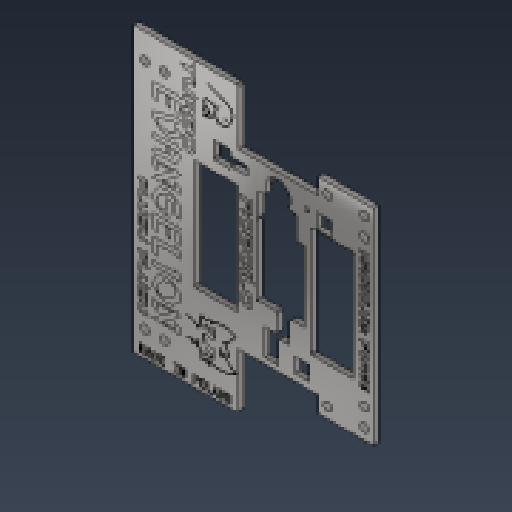
# Autodesk Inventor part: ceil
Saved by Autodesk Inventor 2026.2 (Build 302298010, 298A)
## iProperties
Created: 2026-05-14
Part Number: ceil
Material: Steel, Alloy
Document SubType Name: Modeling
Designer: szymo
Density: 7.73 g/cm^3
Appearance: Semi-Polished
Author: szymo
Autodesk Inventor part; units mm, degrees
(part 1 of 7)
ref_plane "YZ Plane" through (0, 0, 0) normal (1, 0, 0) x (0, 1, 0)
ref_plane "XZ Plane" through (0, 0, 0) normal (0, 1, 0) x (-1, 0, 0)
ref_plane "XY Plane" through (0, 0, 0) normal (0, 0, 1) x (1, 0, 0)
sketch "Katze" plane through (0, 0, 0) normal (0, 0, 1) x (1, 0, 0)
  line L0 (230.7163, -61.7099) -> (230.2113, -62.1007)
  line L1 (230.2113, -62.1007) -> (229.7885, -62.4476)
  line L2 (229.7885, -62.4476) -> (229.4229, -62.7723)
  line L3 (229.4229, -62.7723) -> (229.0894, -63.0967)
  line L4 (229.0894, -63.0967) -> (228.5914, -63.6396)
  line L5 (228.5914, -63.6396) -> (228.3777, -63.9055)
  line L6 (228.3777, -63.9055) -> (228.1831, -64.174)
  line L7 (228.1831, -64.174) -> (228.0044, -64.45)
  line L8 (228.0044, -64.45) -> (227.8384, -64.7383)
  line L9 (227.8384, -64.7383) -> (227.5311, -65.3713)
  line L10 (227.5311, -65.3713) -> (227.3292, -65.8056)
  line L11 (227.3292, -65.8056) -> (227.2039, -65.7151)
  line L12 (227.2039, -65.7151) -> (226.9329, -65.4703)
  line L13 (226.9329, -65.4703) -> (226.5687, -65.1387)
  line L14 (226.5687, -65.1387) -> (226.2195, -64.8603)
  line L15 (226.2195, -64.8603) -> (225.8775, -64.6297)
  line L16 (225.8775, -64.6297) -> (225.5347, -64.4416)
  line L17 (225.5347, -64.4416) -> (225.1793, -64.2897)
  line L18 (225.1793, -64.2897) -> (224.8232, -64.1835)
  line L19 (224.8232, -64.1835) -> (224.4342, -64.1159)
  line L20 (224.4342, -64.1159) -> (223.9802, -64.0797)
  line L21 (223.9802, -64.0797) -> (223.4544, -64.053)
  line L22 (223.4544, -64.053) -> (223.4773, -64.4111)
  line L23 (223.4773, -64.4111) -> (223.5225, -64.766)
  line L24 (223.5225, -64.766) -> (223.6106, -65.1265)
  line L25 (223.6106, -65.1265) -> (223.7387, -65.4827)
  line L26 (223.7387, -65.4827) -> (223.904, -65.8247)
  line L27 (223.904, -65.8247) -> (223.8877, -65.8497)
  line L28 (223.8877, -65.8497) -> (223.8303, -65.8894)
  line L29 (223.8303, -65.8894) -> (223.6435, -65.9885)
  line L30 (223.6435, -65.9885) -> (223.4459, -66.0733)
  line L31 (223.4459, -66.0733) -> (223.3401, -66.0952)
  line L32 (223.3401, -66.0952) -> (221.4618, -63.5691)
  line L33 (221.4618, -63.5691) -> (220.9584, -62.9095)
  line L34 (220.9584, -62.9095) -> (220.4035, -62.2123)
  line L35 (220.4035, -62.2123) -> (219.9444, -61.6601)
  line L36 (219.9444, -61.6601) -> (219.7968, -61.4955)
  line L37 (219.7968, -61.4955) -> (219.7282, -61.4355)
  line L38 (219.7282, -61.4355) -> (219.6713, -61.468)
  line L39 (219.6713, -61.468) -> (219.5901, -61.5779)
  line L40 (219.5901, -61.5779) -> (219.3091, -62.1061)
  line L41 (219.3091, -62.1061) -> (218.9264, -62.93)
  line L42 (218.9264, -62.93) -> (218.7721, -63.3113)
  line L43 (218.7721, -63.3113) -> (218.639, -63.6825)
  line L44 (218.639, -63.6825) -> (218.5248, -64.0511)
  line L45 (218.5248, -64.0511) -> (218.4267, -64.425)
  line L46 (218.4267, -64.425) -> (218.269, -65.2189)
  line L47 (218.269, -65.2189) -> (218.231, -65.5313)
  line L48 (218.231, -65.5313) -> (218.2028, -65.9285)
  line L49 (218.2028, -65.9285) -> (218.1766, -66.8586)
  line L50 (218.1766, -66.8586) -> (218.1918, -67.7708)
  line L51 (218.1918, -67.7708) -> (218.2154, -68.1457)
  line L52 (218.2154, -68.1457) -> (218.2499, -68.4269)
  line L53 (218.2499, -68.4269) -> (218.3989, -69.0835)
  line L54 (218.3989, -69.0835) -> (218.4912, -69.3823)
  line L55 (218.4912, -69.3823) -> (218.5957, -69.6623)
  line L56 (218.5957, -69.6623) -> (218.7127, -69.924)
  line L57 (218.7127, -69.924) -> (218.8425, -70.1682)
  line L58 (218.8425, -70.1682) -> (218.9854, -70.3954)
  line L59 (218.9854, -70.3954) -> (219.1415, -70.6062)
  line L60 (219.1415, -70.6062) -> (219.271, -70.77)
  line L61 (219.271, -70.77) -> (219.1072, -70.77)
  line L62 (219.1072, -70.77) -> (218.8635, -70.7572)
  line L63 (218.8635, -70.7572) -> (218.569, -70.7215)
  line L64 (218.569, -70.7215) -> (217.9451, -70.5986)
  line L65 (217.9451, -70.5986) -> (217.6584, -70.5362)
  line L66 (217.6584, -70.5362) -> (217.583, -70.5316)
  line L67 (217.583, -70.5316) -> (217.5489, -70.5453)
  line L68 (217.5489, -70.5453) -> (217.5385, -70.6213)
  line L69 (217.5385, -70.6213) -> (217.5627, -70.7448)
  line L70 (217.5627, -70.7448) -> (217.6191, -70.9048)
  line L71 (217.6191, -70.9048) -> (217.7051, -71.0901)
  line L72 (217.7051, -71.0901) -> (217.8691, -71.383)
  line L73 (217.8691, -71.383) -> (218.0371, -71.6163)
  line L74 (218.0371, -71.6163) -> (218.2371, -71.8246)
  line L75 (218.2371, -71.8246) -> (218.4976, -72.0426)
  line L76 (218.4976, -72.0426) -> (218.8862, -72.3436)
  line L77 (218.8862, -72.3436) -> (218.8138, -72.4617)
  line L78 (218.8138, -72.4617) -> (218.6627, -72.733)
  line L79 (218.6627, -72.733) -> (218.539, -73.0175)
  line L80 (218.539, -73.0175) -> (218.4318, -73.3441)
  line L81 (218.4318, -73.3441) -> (218.33, -73.7418)
  line L82 (218.33, -73.7418) -> (218.2714, -74.0519)
  line L83 (218.2714, -74.0519) -> (218.2694, -74.1303)
  line L84 (218.2694, -74.1303) -> (218.2842, -74.1648)
  line L85 (218.2842, -74.1648) -> (218.4768, -74.2085)
  line L86 (218.4768, -74.2085) -> (218.8305, -74.2433)
  line L87 (218.8305, -74.2433) -> (219.232, -74.2617)
  line L88 (219.232, -74.2617) -> (219.5682, -74.2562)
  line L89 (219.5682, -74.2562) -> (219.983, -74.2271)
  line L90 (219.983, -74.2271) -> (220.255, -74.2405)
  line L91 (220.255, -74.2405) -> (220.5112, -74.3189)
  line L92 (220.5112, -74.3189) -> (220.8788, -74.4848)
  line L93 (220.8788, -74.4848) -> (221.4389, -74.7477)
  line L94 (221.4389, -74.7477) -> (221.4389, -74.8848)
  line L95 (221.4389, -74.8848) -> (221.4613, -75.0263)
  line L96 (221.4613, -75.0263) -> (221.5151, -75.182)
  line L97 (221.5151, -75.182) -> (221.6288, -75.3502)
  line L98 (221.6288, -75.3502) -> (221.8328, -75.5845)
  line L99 (221.8328, -75.5845) -> (222.0847, -75.8394)
  line L100 (222.0847, -75.8394) -> (222.3419, -76.0698)
  line L101 (222.3419, -76.0698) -> (222.5019, -76.2031)
  line L102 (222.5019, -76.2031) -> (222.3457, -76.3707)
  line L103 (222.3457, -76.3707) -> (222.0391, -76.7223)
  line L104 (222.0391, -76.7223) -> (221.8242, -76.9975)
  line L105 (221.8242, -76.9975) -> (221.7044, -77.1926)
  line L106 (221.7044, -77.1926) -> (221.6811, -77.2591)
  line L107 (221.6811, -77.2591) -> (221.6828, -77.3042)
  line L108 (221.6828, -77.3042) -> (221.7073, -77.3377)
  line L109 (221.7073, -77.3377) -> (221.754, -77.3666)
  line L110 (221.754, -77.3666) -> (221.9066, -77.4094)
  line L111 (221.9066, -77.4094) -> (222.1264, -77.4301)
  line L112 (222.1264, -77.4301) -> (222.399, -77.4261)
  line L113 (222.399, -77.4261) -> (222.7648, -77.4071)
  line L114 (222.7648, -77.4071) -> (222.6695, -77.6204)
  line L115 (222.6695, -77.6204) -> (222.5605, -77.9352)
  line L116 (222.5605, -77.9352) -> (222.4257, -78.39)
  line L117 (222.4257, -78.39) -> (222.2543, -79.0073)
  line L118 (222.2543, -79.0073) -> (222.2504, -79.0421)
  line L119 (222.2504, -79.0421) -> (222.2666, -79.063)
  line L120 (222.2666, -79.063) -> (222.3876, -79.0758)
  line L121 (222.3876, -79.0758) -> (222.5114, -79.0616)
  line L122 (222.5114, -79.0616) -> (222.5366, -79.0405)
  line L123 (222.5366, -79.0405) -> (222.5438, -79.0073)
  line L124 (222.5438, -79.0073) -> (222.5926, -78.7712)
  line L125 (222.5926, -78.7712) -> (222.7086, -78.3591)
  line L126 (222.7086, -78.3591) -> (222.846, -77.9234)
  line L127 (222.846, -77.9234) -> (222.9591, -77.6166)
  line L128 (222.9591, -77.6166) -> (223.0622, -77.3453)
  line L129 (223.0622, -77.3453) -> (223.069, -77.2591)
  line L130 (223.069, -77.2591) -> (223.0405, -77.2004)
  line L131 (223.0405, -77.2004) -> (222.9726, -77.1648)
  line L132 (222.9726, -77.1648) -> (222.8611, -77.1483)
  line L133 (222.8611, -77.1483) -> (222.4905, -77.1556)
  line L134 (222.4905, -77.1556) -> (222.1666, -77.1661)
  line L135 (222.1666, -77.1661) -> (222.0485, -77.148)
  line L136 (222.0485, -77.148) -> (222.1, -77.0622)
  line L137 (222.1, -77.0622) -> (222.2371, -76.8932)
  line L138 (222.2371, -76.8932) -> (222.6657, -76.4241)
  line L139 (222.6657, -76.4241) -> (222.8905, -76.1917)
  line L140 (222.8905, -76.1917) -> (222.6124, -75.9516)
  line L141 (222.6124, -75.9516) -> (222.08, -75.4649)
  line L142 (222.08, -75.4649) -> (221.9223, -75.2959)
  line L143 (221.9223, -75.2959) -> (221.8161, -75.1554)
  line L144 (221.8161, -75.1554) -> (221.7421, -75.0216)
  line L145 (221.7421, -75.0216) -> (221.7094, -74.9229)
  line L146 (221.7094, -74.9229) -> (221.7197, -74.8671)
  line L147 (221.7197, -74.8671) -> (221.7742, -74.862)
  line L148 (221.7742, -74.862) -> (222.1173, -74.9538)
  line L149 (222.1173, -74.9538) -> (222.4705, -75.0311)
  line L150 (222.4705, -75.0311) -> (223.2639, -75.1515)
  line L151 (223.2639, -75.1515) -> (223.4703, -75.1708)
  line L152 (223.4703, -75.1708) -> (223.5863, -75.1601)
  line L153 (223.5863, -75.1601) -> (223.6184, -75.1408)
  line L154 (223.6184, -75.1408) -> (223.6373, -75.1108)
  line L155 (223.6373, -75.1108) -> (223.6487, -75.0144)
  line L156 (223.6487, -75.0144) -> (223.6381, -74.9685)
  line L157 (223.6381, -74.9685) -> (223.5897, -74.9387)
  line L158 (223.5897, -74.9387) -> (223.2791, -74.8887)
  line L159 (223.2791, -74.8887) -> (222.5987, -74.7855)
  line L160 (222.5987, -74.7855) -> (222.0247, -74.6496)
  line L161 (222.0247, -74.6496) -> (221.4521, -74.4493)
  line L162 (221.4521, -74.4493) -> (220.776, -74.1533)
  line L163 (220.776, -74.1533) -> (220.4954, -74.0263)
  line L164 (220.4954, -74.0263) -> (220.3202, -73.9604)
  line L165 (220.3202, -73.9604) -> (220.1957, -73.9395)
  line L166 (220.1957, -73.9395) -> (220.0673, -73.9476)
  line L167 (220.0673, -73.9476) -> (219.402, -74)
  line L168 (219.402, -74) -> (218.9053, -73.9895)
  line L169 (218.9053, -73.9895) -> (218.5738, -73.9628)
  line L170 (218.5738, -73.9628) -> (218.5967, -73.7799)
  line L171 (218.5967, -73.7799) -> (218.6544, -73.5137)
  line L172 (218.6544, -73.5137) -> (218.7557, -73.207)
  line L173 (218.7557, -73.207) -> (218.887, -72.8954)
  line L174 (218.887, -72.8954) -> (219.0348, -72.6141)
  line L175 (219.0348, -72.6141) -> (219.2291, -72.275)
  line L176 (219.2291, -72.275) -> (218.9015, -72.0273)
  line L177 (218.9015, -72.0273) -> (218.6094, -71.801)
  line L178 (218.6094, -71.801) -> (218.3738, -71.5854)
  line L179 (218.3738, -71.5854) -> (218.1867, -71.3726)
  line L180 (218.1867, -71.3726) -> (218.0404, -71.1549)
  line L181 (218.0404, -71.1549) -> (217.9109, -70.8958)
  line L182 (217.9109, -70.8958) -> (218.2614, -70.9415)
  line L183 (218.2614, -70.9415) -> (218.6548, -70.992)
  line L184 (218.6548, -70.992) -> (219.1224, -71.0253)
  line L185 (219.1224, -71.0253) -> (219.5611, -71.0334)
  line L186 (219.5611, -71.0334) -> (219.6405, -71.0183)
  line L187 (219.6405, -71.0183) -> (219.6711, -70.9872)
  line L188 (219.6711, -70.9872) -> (219.6613, -70.9324)
  line L189 (219.6613, -70.9324) -> (219.6101, -70.832)
  line L190 (219.6101, -70.832) -> (219.3891, -70.4995)
  line L191 (219.3891, -70.4995) -> (219.1463, -70.1365)
  line L192 (219.1463, -70.1365) -> (218.9468, -69.7866)
  line L193 (218.9468, -69.7866) -> (218.7866, -69.4362)
  line L194 (218.7866, -69.4362) -> (218.6619, -69.0713)
  line L195 (218.6619, -69.0713) -> (218.5688, -68.6779)
  line L196 (218.5688, -68.6779) -> (218.5035, -68.2423)
  line L197 (218.5035, -68.2423) -> (218.462, -67.7505)
  line L198 (218.462, -67.7505) -> (218.4404, -67.1886)
  line L199 (218.4404, -67.1886) -> (218.4368, -66.5988)
  line L200 (218.4368, -66.5988) -> (218.4554, -66.0518)
  line L201 (218.4554, -66.0518) -> (218.4978, -65.5384)
  line L202 (218.4978, -65.5384) -> (218.5657, -65.0493)
  line L203 (218.5657, -65.0493) -> (218.6605, -64.5752)
  line L204 (218.6605, -64.5752) -> (218.7839, -64.1068)
  line L205 (218.7839, -64.1068) -> (218.9373, -63.6349)
  line L206 (218.9373, -63.6349) -> (219.1224, -63.15)
  line L207 (219.1224, -63.15) -> (219.4782, -62.3623)
  line L208 (219.4782, -62.3623) -> (219.6534, -62.0045)
  line L209 (219.6534, -62.0045) -> (219.7397, -61.8546)
  line L210 (219.7397, -61.8546) -> (220.1416, -62.3123)
  line L211 (220.1416, -62.3123) -> (220.7722, -63.0929)
  line L212 (220.7722, -63.0929) -> (221.2246, -63.6858)
  line L213 (221.2246, -63.6858) -> (221.8199, -64.4988)
  line L214 (221.8199, -64.4988) -> (222.7076, -65.6951)
  line L215 (222.7076, -65.6951) -> (222.9471, -66.0106)
  line L216 (222.9471, -66.0106) -> (223.0634, -66.1818)
  line L217 (223.0634, -66.1818) -> (223.0875, -66.263)
  line L218 (223.0875, -66.263) -> (223.0505, -66.3085)
  line L219 (223.0505, -66.3085) -> (222.7648, -66.5257)
  line L220 (222.7648, -66.5257) -> (222.6237, -66.6473)
  line L221 (222.6237, -66.6473) -> (222.5276, -66.7586)
  line L222 (222.5276, -66.7586) -> (222.4787, -66.8563)
  line L223 (222.4787, -66.8563) -> (222.479, -66.9372)
  line L224 (222.479, -66.9372) -> (222.5372, -66.99)
  line L225 (222.5372, -66.99) -> (222.6467, -67.0401)
  line L226 (222.6467, -67.0401) -> (222.9417, -67.0773)
  line L227 (222.9417, -67.0773) -> (223.4554, -67.101)
  line L228 (223.4554, -67.101) -> (224.0419, -67.1076)
  line L229 (224.0419, -67.1076) -> (224.5555, -67.0934)
  line L230 (224.5555, -67.0934) -> (224.9822, -67.0667)
  line L231 (224.9822, -67.0667) -> (224.9822, -66.941)
  line L232 (224.9822, -66.941) -> (224.9822, -66.8153)
  line L233 (224.9822, -66.8153) -> (224.003, -66.8343)
  line L234 (224.003, -66.8343) -> (223.2744, -66.8381)
  line L235 (223.2744, -66.8381) -> (222.9286, -66.8191)
  line L236 (222.9286, -66.8191) -> (222.889, -66.7928)
  line L237 (222.889, -66.7928) -> (222.9091, -66.7519)
  line L238 (222.9091, -66.7519) -> (223.2068, -66.5448)
  line L239 (223.2068, -66.5448) -> (223.5701, -66.3285)
  line L240 (223.5701, -66.3285) -> (223.9307, -66.1409)
  line L241 (223.9307, -66.1409) -> (224.2888, -65.9733)
  line L242 (224.2888, -65.9733) -> (224.1173, -65.6456)
  line L243 (224.1173, -65.6456) -> (223.9726, -65.3486)
  line L244 (223.9726, -65.3486) -> (223.8707, -65.0898)
  line L245 (223.8707, -65.0898) -> (223.8045, -64.8489)
  line L246 (223.8045, -64.8489) -> (223.7668, -64.6055)
  line L247 (223.7668, -64.6055) -> (223.7402, -64.3311)
  line L248 (223.7402, -64.3311) -> (223.8964, -64.3311)
  line L249 (223.8964, -64.3311) -> (224.1248, -64.3441)
  line L250 (224.1248, -64.3441) -> (224.4064, -64.3773)
  line L251 (224.4064, -64.3773) -> (224.9022, -64.4721)
  line L252 (224.9022, -64.4721) -> (225.1239, -64.5453)
  line L253 (225.1239, -64.5453) -> (225.3466, -64.6395)
  line L254 (225.3466, -64.6395) -> (225.5716, -64.7553)
  line L255 (225.5716, -64.7553) -> (225.7999, -64.8936)
  line L256 (225.7999, -64.8936) -> (226.2711, -65.2399)
  line L257 (226.2711, -65.2399) -> (226.7691, -65.6837)
  line L258 (226.7691, -65.6837) -> (227.0766, -65.969)
  line L259 (227.0766, -65.969) -> (227.2777, -66.1228)
  line L260 (227.2777, -66.1228) -> (227.3484, -66.1562)
  line L261 (227.3484, -66.1562) -> (227.4045, -66.1638)
  line L262 (227.4045, -66.1638) -> (227.4501, -66.1477)
  line L263 (227.4501, -66.1477) -> (227.4892, -66.1104)
  line L264 (227.4892, -66.1104) -> (227.6873, -65.6837)
  line L265 (227.6873, -65.6837) -> (227.8878, -65.2383)
  line L266 (227.8878, -65.2383) -> (228.0964, -64.8312)
  line L267 (228.0964, -64.8312) -> (228.3191, -64.4541)
  line L268 (228.3191, -64.4541) -> (228.5622, -64.0987)
  line L269 (228.5622, -64.0987) -> (228.8319, -63.757)
  line L270 (228.8319, -63.757) -> (229.1345, -63.4205)
  line L271 (229.1345, -63.4205) -> (229.476, -63.0813)
  line L272 (229.476, -63.0813) -> (229.8628, -62.7309)
  line L273 (229.8628, -62.7309) -> (230.2574, -62.4007)
  line L274 (230.2574, -62.4007) -> (230.6534, -62.0923)
  line L275 (230.6534, -62.0923) -> (230.9665, -61.8689)
  line L276 (230.9665, -61.8689) -> (231.0657, -61.8088)
  line L277 (231.0657, -61.8088) -> (231.1125, -61.7937)
  line L278 (231.1125, -61.7937) -> (231.1868, -61.9099)
  line L279 (231.1868, -61.9099) -> (231.3068, -62.1518)
  line L280 (231.3068, -62.1518) -> (231.5392, -62.6918)
  line L281 (231.5392, -62.6918) -> (231.7226, -63.2253)
  line L282 (231.7226, -63.2253) -> (231.8667, -63.786)
  line L283 (231.8667, -63.786) -> (231.9812, -64.4073)
  line L284 (231.9812, -64.4073) -> (232.0137, -64.7027)
  line L285 (232.0137, -64.7027) -> (232.0369, -65.0916)
  line L286 (232.0369, -65.0916) -> (232.0555, -66.0294)
  line L287 (232.0555, -66.0294) -> (232.0369, -66.9802)
  line L288 (232.0369, -66.9802) -> (232.0137, -67.3851)
  line L289 (232.0137, -67.3851) -> (231.9812, -67.703)
  line L290 (231.9812, -67.703) -> (231.9025, -68.1853)
  line L291 (231.9025, -68.1853) -> (231.8111, -68.5999)
  line L292 (231.8111, -68.5999) -> (231.701, -68.9584)
  line L293 (231.701, -68.9584) -> (231.5664, -69.2722)
  line L294 (231.5664, -69.2722) -> (231.4012, -69.553)
  line L295 (231.4012, -69.553) -> (231.1995, -69.8124)
  line L296 (231.1995, -69.8124) -> (230.9554, -70.0618)
  line L297 (230.9554, -70.0618) -> (230.6629, -70.3128)
  line L298 (230.6629, -70.3128) -> (230.3543, -70.5605)
  line L299 (230.3543, -70.5605) -> (231.1506, -70.5795)
  line L300 (231.1506, -70.5795) -> (231.7202, -70.6005)
  line L301 (231.7202, -70.6005) -> (231.9698, -70.6215)
  line L302 (231.9698, -70.6215) -> (231.9636, -70.6739)
  line L303 (231.9636, -70.6739) -> (231.8992, -70.7768)
  line L304 (231.8992, -70.7768) -> (231.6278, -71.0987)
  line L305 (231.6278, -71.0987) -> (231.2207, -71.5162)
  line L306 (231.2207, -71.5162) -> (230.7429, -71.9588)
  line L307 (230.7429, -71.9588) -> (230.541, -72.1378)
  line L308 (230.541, -72.1378) -> (230.8344, -72.5112)
  line L309 (230.8344, -72.5112) -> (231.0881, -72.8489)
  line L310 (231.0881, -72.8489) -> (231.3268, -73.1923)
  line L311 (231.3268, -73.1923) -> (231.5041, -73.4713)
  line L312 (231.5041, -73.4713) -> (231.5735, -73.6161)
  line L313 (231.5735, -73.6161) -> (231.5446, -73.6548)
  line L314 (231.5446, -73.6548) -> (231.4478, -73.6942)
  line L315 (231.4478, -73.6942) -> (230.9906, -73.7952)
  line L316 (230.9906, -73.7952) -> (230.6352, -73.8548)
  line L317 (230.6352, -73.8548) -> (230.3362, -73.8804)
  line L318 (230.3362, -73.8804) -> (230.0615, -73.8739)
  line L319 (230.0615, -73.8739) -> (229.779, -73.8371)
  line L320 (229.779, -73.8371) -> (229.4094, -73.7761)
  line L321 (229.4094, -73.7761) -> (228.9599, -74.0047)
  line L322 (228.9599, -74.0047) -> (228.4698, -74.221)
  line L323 (228.4698, -74.221) -> (227.9312, -74.42)
  line L324 (227.9312, -74.42) -> (227.2911, -74.6448)
  line L325 (227.2911, -74.6448) -> (227.2663, -74.6681)
  line L326 (227.2663, -74.6681) -> (227.2701, -74.7053)
  line L327 (227.2701, -74.7053) -> (227.3863, -74.8658)
  line L328 (227.3863, -74.8658) -> (227.703, -75.2598)
  line L329 (227.703, -75.2598) -> (227.9805, -75.6335)
  line L330 (227.9805, -75.6335) -> (228.2213, -75.9913)
  line L331 (228.2213, -75.9913) -> (228.4279, -76.3379)
  line L332 (228.4279, -76.3379) -> (228.6029, -76.6779)
  line L333 (228.6029, -76.6779) -> (228.7488, -77.0159)
  line L334 (228.7488, -77.0159) -> (228.8682, -77.3565)
  line L335 (228.8682, -77.3565) -> (228.9637, -77.7042)
  line L336 (228.9637, -77.7042) -> (229.0842, -78.4153)
  line L337 (229.0842, -78.4153) -> (229.1732, -79.0606)
  line L338 (229.1732, -79.0606) -> (229.3066, -79.0758)
  line L339 (229.3066, -79.0758) -> (229.384, -79.0733)
  line L340 (229.384, -79.0733) -> (229.4228, -79.0587)
  line L341 (229.4228, -79.0587) -> (229.433, -79.0212)
  line L342 (229.433, -79.0212) -> (229.4247, -78.9501)
  line L343 (229.4247, -78.9501) -> (229.3637, -78.4662)
  line L344 (229.3637, -78.4662) -> (229.2948, -78.0083)
  line L345 (229.2948, -78.0083) -> (229.1936, -77.5604)
  line L346 (229.1936, -77.5604) -> (229.0601, -77.1225)
  line L347 (229.0601, -77.1225) -> (228.8941, -76.6946)
  line L348 (228.8941, -76.6946) -> (228.6957, -76.2767)
  line L349 (228.6957, -76.2767) -> (228.4647, -75.8688)
  line L350 (228.4647, -75.8688) -> (228.201, -75.4709)
  line L351 (228.201, -75.4709) -> (227.9045, -75.083)
  line L352 (227.9045, -75.083) -> (227.6911, -74.7934)
  line L353 (227.6911, -74.7934) -> (228.1826, -74.6181)
  line L354 (228.1826, -74.6181) -> (228.6365, -74.4453)
  line L355 (228.6365, -74.4453) -> (229.0589, -74.2524)
  line L356 (229.0589, -74.2524) -> (229.4552, -74.0428)
  line L357 (229.4552, -74.0428) -> (229.6685, -74.0924)
  line L358 (229.6685, -74.0924) -> (229.9425, -74.1268)
  line L359 (229.9425, -74.1268) -> (230.2857, -74.1338)
  line L360 (230.2857, -74.1338) -> (230.649, -74.1143)
  line L361 (230.649, -74.1143) -> (230.983, -74.0695)
  line L362 (230.983, -74.0695) -> (231.5673, -73.9371)
  line L363 (231.5673, -73.9371) -> (231.9431, -73.8219)
  line L364 (231.9431, -73.8219) -> (231.9467, -73.78)
  line L365 (231.9467, -73.78) -> (231.9126, -73.6867)
  line L366 (231.9126, -73.6867) -> (231.7531, -73.3837)
  line L367 (231.7531, -73.3837) -> (231.5086, -72.9893)
  line L368 (231.5086, -72.9893) -> (231.223, -72.5798)
  line L369 (231.223, -72.5798) -> (230.922, -72.1759)
  line L370 (230.922, -72.1759) -> (231.4707, -71.6349)
  line L371 (231.4707, -71.6349) -> (231.9002, -71.1863)
  line L372 (231.9002, -71.1863) -> (232.1641, -70.8691)
  line L373 (232.1641, -70.8691) -> (232.2545, -70.7041)
  line L374 (232.2545, -70.7041) -> (232.3017, -70.5634)
  line L375 (232.3017, -70.5634) -> (232.3039, -70.4555)
  line L376 (232.3039, -70.4555) -> (232.2876, -70.4165)
  line L377 (232.2876, -70.4165) -> (232.2593, -70.389)
  line L378 (232.2593, -70.389) -> (232.0892, -70.3566)
  line L379 (232.0892, -70.3566) -> (231.7726, -70.3324)
  line L380 (231.7726, -70.3324) -> (231.4374, -70.3231)
  line L381 (231.4374, -70.3231) -> (231.2116, -70.3357)
  line L382 (231.2116, -70.3357) -> (231.0592, -70.3624)
  line L383 (231.0592, -70.3624) -> (231.3068, -70.0957)
  line L384 (231.3068, -70.0957) -> (231.4913, -69.8805)
  line L385 (231.4913, -69.8805) -> (231.6521, -69.6541)
  line L386 (231.6521, -69.6541) -> (231.7914, -69.4103)
  line L387 (231.7914, -69.4103) -> (231.9117, -69.1432)
  line L388 (231.9117, -69.1432) -> (232.0151, -68.8468)
  line L389 (232.0151, -68.8468) -> (232.1041, -68.5151)
  line L390 (232.1041, -68.5151) -> (232.1809, -68.1422)
  line L391 (232.1809, -68.1422) -> (232.2479, -67.722)
  line L392 (232.2479, -67.722) -> (232.2791, -67.4104)
  line L393 (232.2791, -67.4104) -> (232.3015, -67.0096)
  line L394 (232.3015, -67.0096) -> (232.3193, -66.0604)
  line L395 (232.3193, -66.0604) -> (232.3015, -65.1133)
  line L396 (232.3015, -65.1133) -> (232.2791, -64.7153)
  line L397 (232.2791, -64.7153) -> (232.2479, -64.4073)
  line L398 (232.2479, -64.4073) -> (232.174, -63.9707)
  line L399 (232.174, -63.9707) -> (232.0769, -63.5263)
  line L400 (232.0769, -63.5263) -> (231.9634, -63.1032)
  line L401 (231.9634, -63.1032) -> (231.8402, -62.7309)
  line L402 (231.8402, -62.7309) -> (231.6943, -62.3761)
  line L403 (231.6943, -62.3761) -> (231.4954, -61.9385)
  line L404 (231.4954, -61.9385) -> (231.3109, -61.5608)
  line L405 (231.3109, -61.5608) -> (231.2078, -61.386)
  line L406 (231.2078, -61.386) -> (231.0492, -61.4736)
  line L407 (231.0492, -61.4736) -> (230.7163, -61.7099)
  line L408 (227.3368, -69.2727) -> (226.2014, -69.2841)
  line L409 (226.2014, -69.2841) -> (226.2014, -70.1338)
  line L410 (226.2014, -70.1338) -> (226.2243, -71.1244)
  line L411 (226.2243, -71.1244) -> (226.2828, -71.3127)
  line L412 (226.2828, -71.3127) -> (226.3867, -71.4939)
  line L413 (226.3867, -71.4939) -> (226.5227, -71.6494)
  line L414 (226.5227, -71.6494) -> (226.6777, -71.7606)
  line L415 (226.6777, -71.7606) -> (226.825, -71.8199)
  line L416 (226.825, -71.8199) -> (226.9801, -71.8528)
  line L417 (226.9801, -71.8528) -> (227.1376, -71.8603)
  line L418 (227.1376, -71.8603) -> (227.2916, -71.8435)
  line L419 (227.2916, -71.8435) -> (227.4364, -71.8035)
  line L420 (227.4364, -71.8035) -> (227.5665, -71.7414)
  line L421 (227.5665, -71.7414) -> (227.6762, -71.6581)
  line L422 (227.6762, -71.6581) -> (227.7597, -71.5549)
  line L423 (227.7597, -71.5549) -> (227.8665, -71.347)
  line L424 (227.8665, -71.347) -> (227.9307, -71.1063)
  line L425 (227.9307, -71.1063) -> (227.9628, -70.7727)
  line L426 (227.9628, -70.7727) -> (227.9731, -70.2862)
  line L427 (227.9731, -70.2862) -> (227.9731, -69.5547)
  line L428 (227.9731, -69.5547) -> (228.2017, -69.5318)
  line L429 (228.2017, -69.5318) -> (228.4179, -69.5175)
  line L430 (228.4179, -69.5175) -> (228.617, -69.5204)
  line L431 (228.617, -69.5204) -> (228.7227, -69.5302)
  line L432 (228.7227, -69.5302) -> (228.786, -69.5537)
  line L433 (228.786, -69.5537) -> (228.8286, -69.6072)
  line L434 (228.8286, -69.6072) -> (228.8722, -69.7071)
  line L435 (228.8722, -69.7071) -> (228.9364, -69.9068)
  line L436 (228.9364, -69.9068) -> (228.9883, -70.1384)
  line L437 (228.9883, -70.1384) -> (229.0523, -70.6515)
  line L438 (229.0523, -70.6515) -> (229.0576, -71.1553)
  line L439 (229.0576, -71.1553) -> (229.0363, -71.3752)
  line L440 (229.0363, -71.3752) -> (228.998, -71.5587)
  line L441 (228.998, -71.5587) -> (228.9594, -71.7097)
  line L442 (228.9594, -71.7097) -> (228.9522, -71.7835)
  line L443 (228.9522, -71.7835) -> (229.0856, -71.8216)
  line L444 (229.0856, -71.8216) -> (229.1999, -71.8445)
  line L445 (229.1999, -71.8445) -> (229.2685, -71.5701)
  line L446 (229.2685, -71.5701) -> (229.3003, -71.4117)
  line L447 (229.3003, -71.4117) -> (229.3171, -71.2458)
  line L448 (229.3171, -71.2458) -> (229.3142, -70.7586)
  line L449 (229.3142, -70.7586) -> (229.2956, -70.4308)
  line L450 (229.2956, -70.4308) -> (229.2623, -70.1619)
  line L451 (229.2623, -70.1619) -> (229.2054, -69.9008)
  line L452 (229.2054, -69.9008) -> (229.1161, -69.5966)
  line L453 (229.1161, -69.5966) -> (229.106, -69.5481)
  line L454 (229.106, -69.5481) -> (229.1327, -69.5232)
  line L455 (229.1327, -69.5232) -> (229.398, -69.5127)
  line L456 (229.398, -69.5127) -> (229.7066, -69.5127)
  line L457 (229.7066, -69.5127) -> (229.7066, -69.3794)
  line L458 (229.7066, -69.3794) -> (229.7066, -69.246)
  line L459 (229.7066, -69.246) -> (229.0894, -69.2537)
  line L460 (229.0894, -69.2537) -> (227.3368, -69.2727)
  line L461 (220.9931, -69.387) -> (220.1435, -69.3984)
  line L462 (220.1435, -69.3984) -> (220.1435, -69.5318)
  line L463 (220.1435, -69.5318) -> (220.1435, -69.6651)
  line L464 (220.1435, -69.6651) -> (220.4293, -69.6651)
  line L465 (220.4293, -69.6651) -> (220.715, -69.6651)
  line L466 (220.715, -69.6651) -> (220.6388, -69.8175)
  line L467 (220.6388, -69.8175) -> (220.5592, -70.0144)
  line L468 (220.5592, -70.0144) -> (220.4993, -70.249)
  line L469 (220.4993, -70.249) -> (220.4615, -70.5108)
  line L470 (220.4615, -70.5108) -> (220.4483, -70.7891)
  line L471 (220.4483, -70.7891) -> (220.4556, -71.0385)
  line L472 (220.4556, -71.0385) -> (220.4812, -71.2525)
  line L473 (220.4812, -71.2525) -> (220.5303, -71.4615)
  line L474 (220.5303, -71.4615) -> (220.6083, -71.6959)
  line L475 (220.6083, -71.6959) -> (220.6883, -71.873)
  line L476 (220.6883, -71.873) -> (220.7241, -71.8963)
  line L477 (220.7241, -71.8963) -> (220.7684, -71.8902)
  line L478 (220.7684, -71.8902) -> (220.8488, -71.8555)
  line L479 (220.8488, -71.8555) -> (220.8808, -71.7959)
  line L480 (220.8808, -71.7959) -> (220.8669, -71.6834)
  line L481 (220.8669, -71.6834) -> (220.8103, -71.4901)
  line L482 (220.8103, -71.4901) -> (220.7336, -71.1968)
  line L483 (220.7336, -71.1968) -> (220.6883, -70.9377)
  line L484 (220.6883, -70.9377) -> (220.6905, -70.6837)
  line L485 (220.6905, -70.6837) -> (220.7317, -70.3919)
  line L486 (220.7317, -70.3919) -> (220.8035, -70.1072)
  line L487 (220.8035, -70.1072) -> (220.8979, -69.8747)
  line L488 (220.8979, -69.8747) -> (221.0008, -69.6842)
  line L489 (221.0008, -69.6842) -> (221.4351, -69.6537)
  line L490 (221.4351, -69.6537) -> (221.9114, -69.6385)
  line L491 (221.9114, -69.6385) -> (221.9292, -69.6674)
  line L492 (221.9292, -69.6674) -> (221.9366, -69.7413)
  line L493 (221.9366, -69.7413) -> (221.919, -70.05)
  line L494 (221.919, -70.05) -> (221.9029, -70.342)
  line L495 (221.9029, -70.342) -> (221.9084, -70.6209)
  line L496 (221.9084, -70.6209) -> (221.9344, -70.8824)
  line L497 (221.9344, -70.8824) -> (221.9799, -71.1225)
  line L498 (221.9799, -71.1225) -> (222.0441, -71.3368)
  line L499 (222.0441, -71.3368) -> (222.1258, -71.5212)
  line L500 (222.1258, -71.5212) -> (222.2241, -71.6715)
  line L501 (222.2241, -71.6715) -> (222.3381, -71.7835)
  line L502 (222.3381, -71.7835) -> (222.4237, -71.8426)
  line L503 (222.4237, -71.8426) -> (222.5057, -71.8759)
  line L504 (222.5057, -71.8759) -> (222.6135, -71.8907)
  line L505 (222.6135, -71.8907) -> (222.7762, -71.894)
  line L506 (222.7762, -71.894) -> (223.0353, -71.8783)
  line L507 (223.0353, -71.8783) -> (223.1138, -71.8538)
  line L508 (223.1138, -71.8538) -> (223.1801, -71.814)
  line L509 (223.1801, -71.814) -> (223.2925, -71.7131)
  line L510 (223.2925, -71.7131) -> (223.3851, -71.5893)
  line L511 (223.3851, -71.5893) -> (223.4593, -71.4362)
  line L512 (223.4593, -71.4362) -> (223.5168, -71.2477)
  line L513 (223.5168, -71.2477) -> (223.5591, -71.0176)
  line L514 (223.5591, -71.0176) -> (223.5878, -70.7397)
  line L515 (223.5878, -70.7397) -> (223.6106, -70.0157)
  line L516 (223.6106, -70.0157) -> (223.6106, -69.3603)
  line L517 (223.6106, -69.3603) -> (222.7267, -69.368)
  line L518 (222.7267, -69.368) -> (220.9931, -69.387)
  line L519 (224.3421, -71.9778) -> (224.2745, -71.99)
  line L520 (224.2745, -71.99) -> (224.2378, -72.0097)
  line L521 (224.2378, -72.0097) -> (224.2248, -72.0459)
  line L522 (224.2248, -72.0459) -> (224.2278, -72.1074)
  line L523 (224.2278, -72.1074) -> (224.2393, -72.2217)
  line L524 (224.2393, -72.2217) -> (224.666, -72.2331)
  line L525 (224.666, -72.2331) -> (225.0889, -72.2483)
  line L526 (225.0889, -72.2483) -> (225.108, -72.1455)
  line L527 (225.108, -72.1455) -> (225.1146, -72.0688)
  line L528 (225.1146, -72.0688) -> (225.1041, -72.0235)
  line L529 (225.1041, -72.0235) -> (224.9931, -71.9992)
  line L530 (224.9931, -71.9992) -> (224.7703, -71.9807)
  line L531 (224.7703, -71.9807) -> (224.3421, -71.9778)
  line L532 (229.1961, -72.4236) -> (228.9065, -72.7093)
  line L533 (228.9065, -72.7093) -> (228.9065, -72.4845)
  line L534 (228.9065, -72.4845) -> (228.8918, -72.2959)
  line L535 (228.8918, -72.2959) -> (228.8696, -72.2499)
  line L536 (228.8696, -72.2499) -> (228.8341, -72.2217)
  line L537 (228.8341, -72.2217) -> (228.7894, -72.2074)
  line L538 (228.7894, -72.2074) -> (228.7332, -72.2188)
  line L539 (228.7332, -72.2188) -> (228.5408, -72.336)
  line L540 (228.5408, -72.336) -> (228.1941, -72.5684)
  line L541 (228.1941, -72.5684) -> (228.1112, -72.6221)
  line L542 (228.1112, -72.6221) -> (228.0769, -72.6636)
  line L543 (228.0769, -72.6636) -> (228.0869, -72.7109)
  line L544 (228.0869, -72.7109) -> (228.1369, -72.7817)
  line L545 (228.1369, -72.7817) -> (228.2055, -72.8694)
  line L546 (228.2055, -72.8694) -> (228.4188, -72.7131)
  line L547 (228.4188, -72.7131) -> (228.6551, -72.5607)
  line L548 (228.6551, -72.5607) -> (228.6708, -72.6203)
  line L549 (228.6708, -72.6203) -> (228.6779, -72.7627)
  line L550 (228.6779, -72.7627) -> (228.687, -72.8985)
  line L551 (228.687, -72.8985) -> (228.716, -72.9894)
  line L552 (228.716, -72.9894) -> (228.7679, -73.0402)
  line L553 (228.7679, -73.0402) -> (228.8456, -73.056)
  line L554 (228.8456, -73.056) -> (228.9971, -72.9466)
  line L555 (228.9971, -72.9466) -> (229.2637, -72.7008)
  line L556 (229.2637, -72.7008) -> (229.5174, -72.442)
  line L557 (229.5174, -72.442) -> (229.6304, -72.294)
  line L558 (229.6304, -72.294) -> (229.558, -72.2026)
  line L559 (229.558, -72.2026) -> (229.5117, -72.1712)
  line L560 (229.5117, -72.1712) -> (229.4556, -72.1859)
  line L561 (229.4556, -72.1859) -> (229.1961, -72.4236)
  line L562 (220.315, -72.2712) -> (220.0292, -72.3893)
  line L563 (220.0292, -72.3893) -> (219.7216, -72.5879)
  line L564 (219.7216, -72.5879) -> (219.5888, -72.6931)
  line L565 (219.5888, -72.6931) -> (219.5339, -72.7551)
  line L566 (219.5339, -72.7551) -> (219.6025, -72.8655)
  line L567 (219.6025, -72.8655) -> (219.6711, -72.9494)
  line L568 (219.6711, -72.9494) -> (219.8387, -72.8084)
  line L569 (219.8387, -72.8084) -> (220.1011, -72.6222)
  line L570 (220.1011, -72.6222) -> (220.1961, -72.5775)
  line L571 (220.1961, -72.5775) -> (220.2464, -72.576)
  line L572 (220.2464, -72.576) -> (220.2445, -72.6536)
  line L573 (220.2445, -72.6536) -> (220.2083, -72.8084)
  line L574 (220.2083, -72.8084) -> (220.1764, -72.9417)
  line L575 (220.1764, -72.9417) -> (220.1691, -73.0391)
  line L576 (220.1691, -73.0391) -> (220.19, -73.101)
  line L577 (220.19, -73.101) -> (220.2431, -73.128)
  line L578 (220.2431, -73.128) -> (220.332, -73.1205)
  line L579 (220.332, -73.1205) -> (220.4606, -73.079)
  line L580 (220.4606, -73.079) -> (220.8522, -72.896)
  line L581 (220.8522, -72.896) -> (221.317, -72.6598)
  line L582 (221.317, -72.6598) -> (221.2637, -72.5531)
  line L583 (221.2637, -72.5531) -> (221.2103, -72.4464)
  line L584 (221.2103, -72.4464) -> (220.8674, -72.6179)
  line L585 (220.8674, -72.6179) -> (220.5017, -72.7893)
  line L586 (220.5017, -72.7893) -> (220.4936, -72.705)
  line L587 (220.4936, -72.705) -> (220.5055, -72.5036)
  line L588 (220.5055, -72.5036) -> (220.5145, -72.3026)
  line L589 (220.5145, -72.3026) -> (220.4978, -72.2217)
  line L590 (220.4978, -72.2217) -> (220.315, -72.2712)
  line L591 (226.3729, -72.9951) -> (226.271, -73.0999)
  line L592 (226.271, -73.0999) -> (226.1633, -73.1703)
  line L593 (226.1633, -73.1703) -> (226.0772, -73.1933)
  line L594 (226.0772, -73.1933) -> (225.9607, -73.2053)
  line L595 (225.9607, -73.2053) -> (225.6656, -73.1989)
  line L596 (225.6656, -73.1989) -> (225.3355, -73.1553)
  line L597 (225.3355, -73.1553) -> (225.0279, -73.0789)
  line L598 (225.0279, -73.0789) -> (224.7155, -72.976)
  line L599 (224.7155, -72.976) -> (224.4755, -73.1437)
  line L600 (224.4755, -73.1437) -> (224.1591, -73.351)
  line L601 (224.1591, -73.351) -> (224.0337, -73.4146)
  line L602 (224.0337, -73.4146) -> (223.9245, -73.4532)
  line L603 (223.9245, -73.4532) -> (223.8272, -73.4679)
  line L604 (223.8272, -73.4679) -> (223.7377, -73.4598)
  line L605 (223.7377, -73.4598) -> (223.6517, -73.4301)
  line L606 (223.6517, -73.4301) -> (223.5649, -73.3799)
  line L607 (223.5649, -73.3799) -> (223.3896, -73.2846)
  line L608 (223.3896, -73.2846) -> (223.3468, -73.3134)
  line L609 (223.3468, -73.3134) -> (223.3068, -73.3804)
  line L610 (223.3068, -73.3804) -> (223.2825, -73.4566)
  line L611 (223.2825, -73.4566) -> (223.2868, -73.5132)
  line L612 (223.2868, -73.5132) -> (223.3743, -73.5827)
  line L613 (223.3743, -73.5827) -> (223.5297, -73.6575)
  line L614 (223.5297, -73.6575) -> (223.7036, -73.7174)
  line L615 (223.7036, -73.7174) -> (223.8468, -73.7418)
  line L616 (223.8468, -73.7418) -> (224.0011, -73.7092)
  line L617 (224.0011, -73.7092) -> (224.2093, -73.6233)
  line L618 (224.2093, -73.6233) -> (224.4324, -73.5024)
  line L619 (224.4324, -73.5024) -> (224.6317, -73.3647)
  line L620 (224.6317, -73.3647) -> (224.7536, -73.2875)
  line L621 (224.7536, -73.2875) -> (224.7967, -73.2768)
  line L622 (224.7967, -73.2768) -> (224.8298, -73.2846)
  line L623 (224.8298, -73.2846) -> (225.0092, -73.3494)
  line L624 (225.0092, -73.3494) -> (225.2823, -73.4142)
  line L625 (225.2823, -73.4142) -> (225.5767, -73.4647)
  line L626 (225.5767, -73.4647) -> (225.8204, -73.4866)
  line L627 (225.8204, -73.4866) -> (226.049, -73.4749)
  line L628 (226.049, -73.4749) -> (226.2314, -73.4304)
  line L629 (226.2314, -73.4304) -> (226.3846, -73.3473)
  line L630 (226.3846, -73.3473) -> (226.5253, -73.2199)
  line L631 (226.5253, -73.2199) -> (226.6148, -73.113)
  line L632 (226.6148, -73.113) -> (226.65, -73.0389)
  line L633 (226.65, -73.0389) -> (226.6324, -72.982)
  line L634 (226.6324, -72.982) -> (226.5634, -72.9265)
  line L635 (226.5634, -72.9265) -> (226.51, -72.8954)
  line L636 (226.51, -72.8954) -> (226.471, -72.8922)
  line L637 (226.471, -72.8922) -> (226.4305, -72.9233)
  line L638 (226.4305, -72.9233) -> (226.3729, -72.9951)
  point P0 (169.824, -150.8274)
sketch "HackClub" plane through (0, 0, 0) normal (0, 0, 1) x (1, 0, 0)
  line L0 (170.4091, 43.542) -> (169.7671, 43.2439)
  line L1 (169.7671, 43.2439) -> (169.2097, 42.9141)
  line L2 (169.2097, 42.9141) -> (168.9319, 42.5807)
  line L3 (168.9319, 42.5807) -> (168.744, 42.2579)
  line L4 (168.744, 42.2579) -> (168.2995, 41.4112)
  line L5 (168.2995, 41.4112) -> (167.7818, 40.3767)
  line L6 (167.7818, 40.3767) -> (167.6, 39.9319)
  line L7 (167.6, 39.9319) -> (167.5023, 39.6121)
  line L8 (167.5023, 39.6121) -> (167.4458, 39.4709)
  line L9 (167.4458, 39.4709) -> (167.1354, 38.8324)
  line L10 (167.1354, 38.8324) -> (166.8038, 38.0246)
  line L11 (166.8038, 38.0246) -> (166.2746, 36.7052)
  line L12 (166.2746, 36.7052) -> (165.689, 35.2235)
  line L13 (165.816, 34.5956) -> (165.9641, 35.0401)
  line L14 (165.9641, 35.0401) -> (166.0231, 35.2636)
  line L15 (166.0231, 35.2636) -> (166.182, 35.6962)
  line L16 (166.182, 35.6962) -> (166.6909, 36.9027)
  line L17 (166.6909, 36.9027) -> (167.093, 37.8905)
  line L18 (167.093, 37.8905) -> (167.4458, 38.7654)
  line L19 (167.4458, 38.7654) -> (167.8762, 39.7884)
  line L20 (167.8762, 39.7884) -> (168.3172, 40.7789)
  line L21 (168.3172, 40.7789) -> (168.8851, 41.8275)
  line L22 (168.8851, 41.8275) -> (169.0651, 42.1538)
  line L23 (169.0651, 42.1538) -> (169.1391, 42.3426)
  line L24 (169.1391, 42.3426) -> (169.201, 42.4776)
  line L25 (169.201, 42.4776) -> (169.3799, 42.6451)
  line L26 (169.3799, 42.6451) -> (169.666, 42.8377)
  line L27 (169.666, 42.8377) -> (170.0493, 43.0481)
  line L28 (170.0493, 43.0481) -> (170.3396, 43.1881)
  line L29 (170.3396, 43.1881) -> (170.5617, 43.2686)
  line L30 (170.5617, 43.2686) -> (170.7746, 43.3041)
  line L31 (170.7746, 43.3041) -> (171.0371, 43.3092)
  line L32 (171.0371, 43.3092) -> (171.6941, 43.2677)
  line L33 (171.6941, 43.2677) -> (172.1025, 43.1892)
  line L34 (172.1025, 43.1892) -> (172.4905, 43.0622)
  line L35 (172.4905, 43.0622) -> (172.9772, 42.856)
  line L36 (172.9772, 42.856) -> (173.5683, 42.5234)
  line L37 (173.5683, 42.5234) -> (174.1356, 42.1444)
  line L38 (174.1356, 42.1444) -> (174.5508, 41.7993)
  line L39 (174.5508, 41.7993) -> (174.8958, 41.417)
  line L40 (174.8958, 41.417) -> (175.1734, 41.0426)
  line L41 (175.1734, 41.0426) -> (175.3743, 40.692)
  line L42 (175.3743, 40.692) -> (175.4892, 40.3811)
  line L43 (175.4892, 40.3811) -> (175.5509, 39.9093)
  line L44 (175.5509, 39.9093) -> (175.602, 39.2099)
  line L45 (175.602, 39.2099) -> (175.6514, 38.3562)
  line L46 (175.6514, 38.3562) -> (175.4609, 38.1727)
  line L47 (175.4609, 38.1727) -> (175.227, 38.02)
  line L48 (175.227, 38.02) -> (174.8647, 37.8508)
  line L49 (174.8647, 37.8508) -> (174.4231, 37.6856)
  line L50 (174.4231, 37.6856) -> (173.951, 37.5448)
  line L51 (173.951, 37.5448) -> (173.5542, 37.4848)
  line L52 (173.5542, 37.4848) -> (173.1044, 37.5095)
  line L53 (173.1044, 37.5095) -> (172.4535, 37.6047)
  line L54 (172.4535, 37.6047) -> (172.1519, 37.7)
  line L55 (172.1519, 37.7) -> (171.7638, 37.8199)
  line L56 (171.7638, 37.8199) -> (171.5748, 37.9012)
  line L57 (171.5748, 37.9012) -> (171.389, 38.0413)
  line L58 (171.389, 38.0413) -> (171.2389, 38.2119)
  line L59 (171.2389, 38.2119) -> (171.157, 38.3844)
  line L60 (171.157, 38.3844) -> (171.0856, 38.5114)
  line L61 (171.0856, 38.5114) -> (170.9665, 38.5537)
  line L62 (170.9665, 38.5537) -> (170.8915, 38.5469)
  line L63 (170.8915, 38.5469) -> (170.8528, 38.5202)
  line L64 (170.8528, 38.5202) -> (170.8607, 38.3703)
  line L65 (170.8607, 38.3703) -> (170.9463, 38.1648)
  line L66 (170.9463, 38.1648) -> (171.0794, 37.9328)
  line L67 (171.0794, 37.9328) -> (171.1713, 37.7902)
  line L68 (171.1713, 37.7902) -> (171.2055, 37.6965)
  line L69 (171.2055, 37.6965) -> (171.1856, 37.6133)
  line L70 (171.1856, 37.6133) -> (171.1147, 37.5024)
  line L71 (171.1147, 37.5024) -> (171.0064, 37.2879)
  line L72 (171.0064, 37.2879) -> (170.8783, 36.9398)
  line L73 (170.8783, 36.9398) -> (170.6631, 36.1548)
  line L74 (170.6631, 36.1548) -> (170.5855, 35.8021)
  line L75 (170.5855, 35.8021) -> (170.5229, 35.3496)
  line L76 (170.5229, 35.3496) -> (170.4444, 34.4262)
  line L77 (170.4444, 34.4262) -> (170.3315, 33.6642)
  line L78 (170.3315, 33.6642) -> (170.3127, 33.4987)
  line L79 (170.3127, 33.4987) -> (170.3501, 33.3723)
  line L80 (170.3501, 33.3723) -> (170.4258, 33.316)
  line L81 (170.4258, 33.316) -> (170.522, 33.3608)
  line L82 (170.522, 33.3608) -> (170.6032, 33.4929)
  line L83 (170.6032, 33.4929) -> (170.6631, 33.7189)
  line L84 (170.6631, 33.7189) -> (170.7619, 34.6379)
  line L85 (170.7619, 34.6379) -> (170.8645, 35.4928)
  line L86 (170.8645, 35.4928) -> (171.0318, 36.3392)
  line L87 (171.0318, 36.3392) -> (171.2283, 37.0281)
  line L88 (171.2283, 37.0281) -> (171.3262, 37.267)
  line L89 (171.3262, 37.267) -> (171.4181, 37.4107)
  line L90 (171.4181, 37.4107) -> (171.5189, 37.4989)
  line L91 (171.5189, 37.4989) -> (171.6051, 37.5342)
  line L92 (171.6051, 37.5342) -> (171.7177, 37.5218)
  line L93 (171.7177, 37.5218) -> (171.8979, 37.4672)
  line L94 (171.8979, 37.4672) -> (172.621, 37.2675)
  line L95 (172.621, 37.2675) -> (173.264, 37.177)
  line L96 (173.264, 37.177) -> (173.8078, 37.1963)
  line L97 (173.8078, 37.1963) -> (174.0365, 37.2473)
  line L98 (174.0365, 37.2473) -> (174.2333, 37.3261)
  line L99 (174.2333, 37.3261) -> (174.4308, 37.3966)
  line L100 (174.4308, 37.3966) -> (174.5543, 37.406)
  line L101 (174.5543, 37.406) -> (174.8471, 37.5086)
  line L102 (174.8471, 37.5086) -> (175.475, 37.8058)
  line L103 (175.475, 37.8058) -> (175.7035, 37.976)
  line L104 (175.7035, 37.976) -> (175.8419, 38.1304)
  line L105 (175.8419, 38.1304) -> (175.8896, 38.4325)
  line L106 (175.8896, 38.4325) -> (175.9054, 38.9859)
  line L107 (175.9054, 38.9859) -> (175.8896, 39.6266)
  line L108 (175.8896, 39.6266) -> (175.8419, 40.1906)
  line L109 (175.8419, 40.1906) -> (175.7595, 40.562)
  line L110 (175.7595, 40.562) -> (175.6162, 40.9182)
  line L111 (175.6162, 40.9182) -> (175.4093, 41.2651)
  line L112 (175.4093, 41.2651) -> (175.1364, 41.6088)
  line L113 (175.1364, 41.6088) -> (174.7602, 42.021)
  line L114 (174.7602, 42.021) -> (174.4555, 42.3135)
  line L115 (174.4555, 42.3135) -> (174.172, 42.5305)
  line L116 (174.172, 42.5305) -> (173.8593, 42.7165)
  line L117 (173.8593, 42.7165) -> (173.3725, 42.9987)
  line L118 (173.3725, 42.9987) -> (173.1696, 43.1274)
  line L119 (173.1696, 43.1274) -> (172.7763, 43.2871)
  line L120 (172.7763, 43.2871) -> (172.293, 43.4402)
  line L121 (172.293, 43.4402) -> (171.8203, 43.5491)
  line L122 (171.8203, 43.5491) -> (171.4182, 43.6035)
  line L123 (171.4182, 43.6035) -> (171.0274, 43.6196)
  line L124 (171.0274, 43.6196) -> (170.6802, 43.5987)
  line L125 (170.6802, 43.5987) -> (170.4091, 43.542)
  line L126 (173.436, 40.875) -> (173.3284, 40.7577)
  line L127 (173.3284, 40.7577) -> (173.3268, 40.7212)
  line L128 (173.3268, 40.7212) -> (173.3584, 40.6986)
  line L129 (173.3584, 40.6986) -> (173.4069, 40.6519)
  line L130 (173.4069, 40.6519) -> (173.4078, 40.5998)
  line L131 (173.4078, 40.5998) -> (173.4254, 40.5231)
  line L132 (173.4254, 40.5231) -> (173.5277, 40.4305)
  line L133 (173.5277, 40.4305) -> (173.6688, 40.3582)
  line L134 (173.6688, 40.3582) -> (173.7162, 40.3809)
  line L135 (173.7162, 40.3809) -> (173.7676, 40.4446)
  line L136 (173.7676, 40.4446) -> (173.8375, 40.5545)
  line L137 (173.8375, 40.5545) -> (173.8558, 40.6519)
  line L138 (173.8558, 40.6519) -> (173.8212, 40.7532)
  line L139 (173.8212, 40.7532) -> (173.7323, 40.875)
  line L140 (173.7323, 40.875) -> (173.5983, 41.0232)
  line L141 (173.5983, 41.0232) -> (173.436, 40.875)
  line L142 (174.8189, 36.3877) -> (174.2685, 35.7315)
  line L143 (174.2685, 35.7315) -> (173.9399, 35.3319)
  line L144 (173.9399, 35.3319) -> (173.5021, 34.8734)
  line L145 (173.5021, 34.8734) -> (171.9049, 33.3961)
  line L146 (171.9049, 33.3961) -> (171.5724, 33.053)
  line L147 (171.5724, 33.053) -> (171.4932, 32.9288)
  line L148 (171.4932, 32.9288) -> (171.4675, 32.8317)
  line L149 (171.4675, 32.8317) -> (171.4816, 32.7179)
  line L150 (171.4816, 32.7179) -> (171.538, 32.7682)
  line L151 (171.538, 32.7682) -> (171.5865, 32.8246)
  line L152 (171.5865, 32.8246) -> (171.6086, 32.8175)
  line L153 (171.6086, 32.8175) -> (171.7047, 32.8555)
  line L154 (171.7047, 32.8555) -> (171.9332, 33.0363)
  line L155 (171.9332, 33.0363) -> (172.2339, 33.2612)
  line L156 (172.2339, 33.2612) -> (172.3509, 33.2952)
  line L157 (172.3509, 33.2952) -> (172.4764, 33.2903)
  line L158 (172.4764, 33.2903) -> (176.0042, 32.8669)
  line L159 (176.0042, 32.8669) -> (176.2388, 32.8564)
  line L160 (176.2388, 32.8564) -> (176.3358, 32.8881)
  line L161 (176.3358, 32.8881) -> (176.2018, 33.2973)
  line L162 (176.2018, 33.2973) -> (176.0695, 33.7127)
  line L163 (176.0695, 33.7127) -> (175.9478, 34.2075)
  line L164 (175.9478, 34.2075) -> (175.7873, 34.8554)
  line L165 (175.7873, 34.8554) -> (175.5738, 35.5595)
  line L166 (175.5738, 35.5595) -> (175.3604, 36.1591)
  line L167 (175.3604, 36.1591) -> (175.1999, 36.4935)
  line L168 (175.1999, 36.4935) -> (175.0729, 36.6628)
  line L169 (175.0729, 36.6628) -> (174.8189, 36.3877)
  line L170 (175.4045, 35.6257) -> (175.8022, 34.1519)
  line L171 (175.8022, 34.1519) -> (175.973, 33.4061)
  line L172 (175.973, 33.4061) -> (176.0254, 33.0645)
  line L173 (176.0254, 33.0645) -> (175.4904, 33.098)
  line L174 (175.4904, 33.098) -> (174.3488, 33.2268)
  line L175 (174.3488, 33.2268) -> (173.1689, 33.382)
  line L176 (173.1689, 33.382) -> (172.5188, 33.4949)
  line L177 (172.5188, 33.4949) -> (172.6881, 33.6889)
  line L178 (172.6881, 33.6889) -> (173.1538, 34.1369)
  line L179 (173.1538, 34.1369) -> (173.9713, 34.9466)
  line L180 (173.9713, 34.9466) -> (174.7836, 35.8938)
  line L181 (174.7836, 35.8938) -> (174.9977, 36.1426)
  line L182 (174.9977, 36.1426) -> (175.0731, 36.1953)
  line L183 (175.0731, 36.1953) -> (175.1364, 36.1963)
  line L184 (175.1364, 36.1963) -> (175.1944, 36.1427)
  line L185 (175.1944, 36.1427) -> (175.2539, 36.0317)
  line L186 (175.2539, 36.0317) -> (175.4045, 35.6257)
  line L187 (174.1839, 34.8566) -> (173.9078, 34.6591)
  line L188 (173.9078, 34.6591) -> (173.7323, 34.5038)
  line L189 (173.7323, 34.5038) -> (173.6589, 34.386)
  line L190 (173.6589, 34.386) -> (173.6626, 34.3576)
  line L191 (173.6626, 34.3576) -> (173.69, 34.3495)
  line L192 (173.69, 34.3495) -> (173.8057, 34.3937)
  line L193 (173.8057, 34.3937) -> (173.9863, 34.5179)
  line L194 (173.9863, 34.5179) -> (174.2544, 34.7296)
  line L195 (174.2544, 34.7296) -> (174.4238, 34.5885)
  line L196 (174.4238, 34.5885) -> (174.5931, 34.4544)
  line L197 (174.5931, 34.4544) -> (174.4449, 34.4121)
  line L198 (174.4449, 34.4121) -> (174.355, 34.3608)
  line L199 (174.355, 34.3608) -> (174.2968, 34.2825)
  line L200 (174.2968, 34.2825) -> (174.2862, 34.2107)
  line L201 (174.2862, 34.2107) -> (174.3391, 34.1793)
  line L202 (174.3391, 34.1793) -> (174.5172, 34.2422)
  line L203 (174.5172, 34.2422) -> (174.7854, 34.3865)
  line L204 (174.7854, 34.3865) -> (175.0297, 34.5454)
  line L205 (175.0297, 34.5454) -> (175.1364, 34.652)
  line L206 (175.1364, 34.652) -> (175.1267, 34.7183)
  line L207 (175.1267, 34.7183) -> (175.0905, 34.7375)
  line L208 (175.0905, 34.7375) -> (174.8965, 34.6379)
  line L209 (174.8965, 34.6379) -> (174.8055, 34.584)
  line L210 (174.8055, 34.584) -> (174.7404, 34.5717)
  line L211 (174.7404, 34.5717) -> (174.6002, 34.6802)
  line L212 (174.6002, 34.6802) -> (174.5181, 34.8063)
  line L213 (174.5181, 34.8063) -> (174.5238, 34.8419)
  line L214 (174.5238, 34.8419) -> (174.5578, 34.8637)
  line L215 (174.5578, 34.8637) -> (174.6139, 34.9148)
  line L216 (174.6139, 34.9148) -> (174.6416, 34.9924)
  line L217 (174.6416, 34.9924) -> (174.6362, 35.0621)
  line L218 (174.6362, 35.0621) -> (174.5931, 35.0894)
  line L219 (174.5931, 35.0894) -> (174.1839, 34.8566)
  line L220 (174.96, 34.1722) -> (174.9565, 34.0214)
  line L221 (174.9565, 34.0214) -> (175.0588, 33.8759)
  line L222 (175.0588, 33.8759) -> (175.1786, 33.786)
  line L223 (175.1786, 33.786) -> (175.2501, 33.7815)
  line L224 (175.2501, 33.7815) -> (175.2542, 33.8471)
  line L225 (175.2542, 33.8471) -> (175.1717, 33.9676)
  line L226 (175.1717, 33.9676) -> (175.0893, 34.0781)
  line L227 (175.0893, 34.0781) -> (175.0843, 34.1422)
  line L228 (175.0843, 34.1422) -> (175.1548, 34.1561)
  line L229 (175.1548, 34.1561) -> (175.2987, 34.1158)
  line L230 (175.2987, 34.1158) -> (175.4415, 34.085)
  line L231 (175.4415, 34.085) -> (175.5209, 34.1078)
  line L232 (175.5209, 34.1078) -> (175.5209, 34.1664)
  line L233 (175.5209, 34.1664) -> (175.4257, 34.2428)
  line L234 (175.4257, 34.2428) -> (175.2646, 34.3052)
  line L235 (175.2646, 34.3052) -> (175.1267, 34.3133)
  line L236 (175.1267, 34.3133) -> (175.0218, 34.2686)
  line L237 (175.0218, 34.2686) -> (174.96, 34.1722)
  point P0 (180.1526, 29.6488)